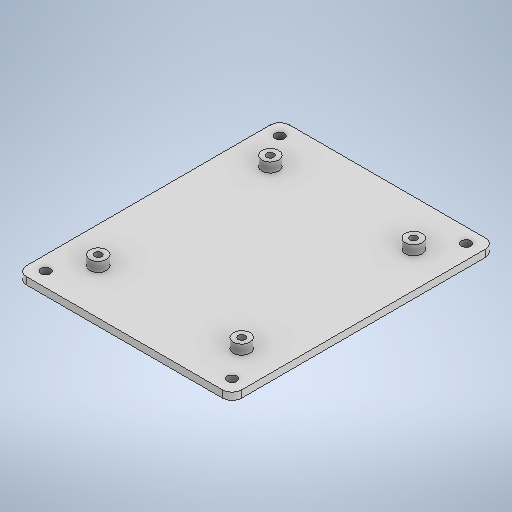
# Autodesk Inventor part: Część1
Saved by Autodesk Inventor 2025.1 (Build 291241000, 241)
## iProperties
Created: 2024-11-12
Part Number: Część1
Material: Ogólny
Document SubType Name: Modeling
Designer: Marek
Density: 1 g/cm^3
Appearance: Domyślna
Author: Marek
Autodesk Inventor part; units mm, degrees
ref_plane "YZ Plane" through (0, 0, 0) normal (1, 0, 0) x (0, 1, 0)
ref_plane "XZ Plane" through (0, 0, 0) normal (0, 1, 0) x (-1, 0, 0)
ref_plane "XY Plane" through (0, 0, 0) normal (0, 0, 1) x (1, 0, 0)
sketch "Szkic1" plane through (0, 0, 0) normal (0, 1, 0) x (-1, 0, 0)
  line L0 (-41, -55) -> (41, -55)
  line L1 (45, -51) -> (45, 51)
  line L2 (41, 55) -> (-41, 55)
  line L3 (-45, 51) -> (-45, -51)
  arc A0 (-41, 55) -> (-45, 51) centre (-41, 51) ccw
  arc A1 (45, 51) -> (41, 55) centre (41, 51) ccw
  arc A2 (41, -55) -> (45, -51) centre (41, -51) ccw
  arc A3 (-45, -51) -> (-41, -55) centre (-41, -51) ccw
  dimension "d14" = 4
  dimension "d15" = 4
  dimension "d16" = 4
  dimension "d17" = 4
  constraints: 8 end point, 8 point on circle, 8 tangent, 4 centre point, 2 parallel, 1 horizontal, 1 perpendicular
  measures "d14" radius of A0
  measures "d15" radius of A1
  measures "d16" radius of A2
  measures "d17" radius of A3
extrude "Wyciągnięcie proste1" add sketch "Szkic1" along normal blind 3
sketch "Szkic2" plane through (0, 3, 0) normal (0, 1, 0) x (1, 0, 0)
  circle A0 centre (-30, -36) radius 1.5
  circle A1 centre (-30, -36) radius 3.5
  circle A2 centre (-30, 36) radius 1.5
  circle A3 centre (-30, 36) radius 3.5
  circle A4 centre (30, -36) radius 1.5
  circle A5 centre (30, -36) radius 3.5
  circle A6 centre (30, 36) radius 1.5
  circle A7 centre (30, 36) radius 3.5
  point P0 (0, 0)
  dimension "d24" = 3
  dimension "d25" = 7
  constraints: 8 centre point, 4 coincident
  measures "d24" diameter of A0
  measures "d25" diameter of A1
extrude "Wyciągnięcie proste2" add sketch "Szkic2" along normal blind 4
sketch "Szkic3" plane through (0, 3, 0) normal (0, 1, 0) x (1, 0, 0)
  circle A0 centre (39, -49) radius 2
  circle A1 centre (-39, -49) radius 2
  circle A2 centre (39, 49) radius 2
  circle A3 centre (-39, 49) radius 2
  point P0 (0, 0)
  dimension "d30" = 4
  constraints: 4 centre point
  measures "d30" diameter of A0
extrude "Wyciągnięcie proste3" cut sketch "Szkic3" against normal through all
thread "Gwint1" size "M4x0.7" class "6H" standard "ISO Metric profile" full length
thread "Gwint2" size "M4x0.7" class "6H" standard "ISO Metric profile" full length
thread "Gwint3" size "M4x0.7" class "6H" standard "ISO Metric profile" full length
thread "Gwint4" size "M4x0.7" class "6H" standard "ISO Metric profile" full length
thread "Gwint5" size "M3x0.5" class "6H" standard "ISO Metric profile" full length
thread "Gwint6" size "M3x0.5" class "6H" standard "ANSI Metric M Profile" full length
thread "Gwint7" size "M3x0.5" class "6H" standard "ANSI Metric M Profile" full length
thread "Gwint8" size "M3x0.5" class "6H" standard "ANSI Metric M Profile" full length
